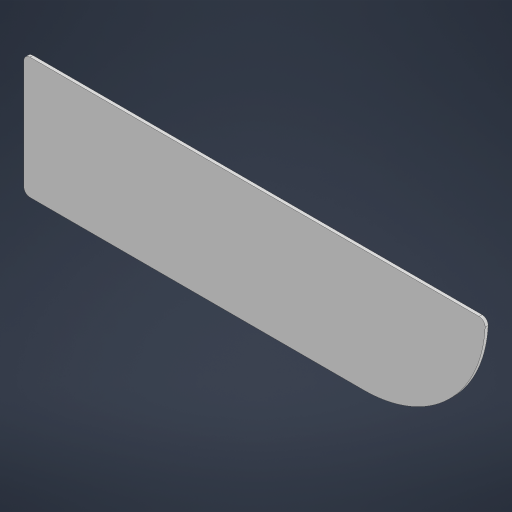
# Autodesk Inventor part: Flaps
Saved by Autodesk Inventor 2023 (Build 270158000, 158)
## iProperties
Created: 2023-11-10
Part Number: Flaps
Material: Generic
Document SubType Name: Modeling
Designer: diego
Density: 1 g/cm^3
Appearance: Default
Author: diego
Autodesk Inventor part; units mm, degrees
ref_plane "YZ Plane" through (0, 0, 0) normal (1, 0, 0) x (0, 1, 0)
ref_plane "XZ Plane" through (0, 0, 0) normal (0, 1, 0) x (-1, 0, 0)
ref_plane "XY Plane" through (0, 0, 0) normal (0, 0, 1) x (1, 0, 0)
sketch "Sketch1" plane through (0, 0, 0) normal (0, 0, 1) x (1, 0, 0)
  arc A0 (0, -63.5) -> (63.5, 0) centre (0, 0) ccw
  line L0 (0, 0) -> (-177.8, 0)
  line L1 (0, -63.5) -> (-177.8, -63.5)
  line L2 (-177.8, 0) -> (-177.8, -63.5)
  line L3 (0, 0) -> (63.5, 0)
  dimension "d0" = 127
  dimension "d1" = 177.8
  dimension "d2" = 177.8
  constraints: 8 end point, 3 horizontal, 2 point on circle, 1 centre point, 1 coincident, 1 point on line, 1 tangent
  measures "d0" diameter of A0
  measures "d1" distance of L0.start L0.end
  measures "d2" distance of L1.start L1.end
extrude "Extrusion1" add sketch "Sketch1" along normal blind 1.5875
fillet "Fillet1" radius 3.175 1 edges at (63.5, 0, 0.7937)
fillet "Fillet2" radius 3.175 1 edges at (-177.8, 0, 0.7937)
fillet "Fillet3" radius 3.175 1 edges at (-177.8, -63.5, 0.7937)
body "Solid1"
